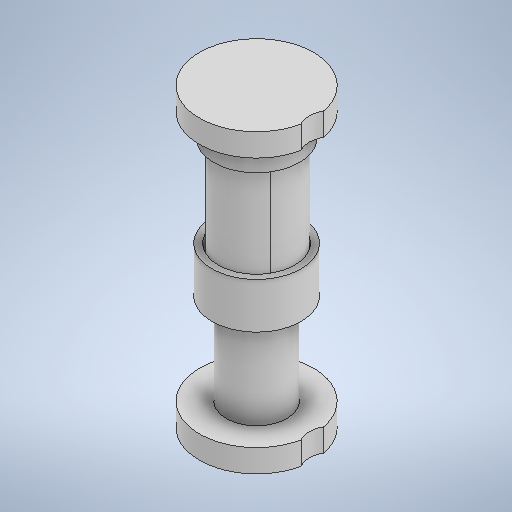
# Autodesk Inventor part: MOULD
Saved by Autodesk Inventor 2026 (Build 300175050, 175E)
## iProperties
Created: 2025-09-13
Part Number: MOULD
Material: Generic
Document SubType Name: Modeling
Designer: Cupri
Density: 1 g/cm^3
Appearance: Default
Author: Cupri
Autodesk Inventor part; units mm, degrees
ref_plane "YZ Plane" through (0, 0, 0) normal (1, 0, 0) x (0, 1, 0)
ref_plane "XZ Plane" through (0, 0, 0) normal (0, 1, 0) x (-1, 0, 0)
ref_plane "XY Plane" through (0, 0, 0) normal (0, 0, 1) x (1, 0, 0)
sketch "Sketch1" plane through (0, 0, 0) normal (0, 1, 0) x (-1, 0, 0)
  circle A0 centre (0, 0) radius 6.75
  circle A1 centre (0, 0) radius 8.25
  dimension "d0" = 13.5
  dimension "d1" = 1.5
  constraints: 2 centre point, 2 coincident
  measures "d0" diameter of A0
  measures "d1" radial gap between concentric circles of A0 A1
extrude "Extrusion1" add sketch "Sketch1" along normal blind 30
sketch "Sketch2" plane through (0, 30, 0) normal (0, 1, 0) x (1, 0, 0)
  circle A0 centre (0, 0) radius 12.5
  dimension "d4" = 25
  constraints: 1 centre point, 1 coincident
  measures "d4" diameter of A0
extrude "Extrusion2" add sketch "Sketch2" along normal blind 5 separate body
sketch "Sketch3" plane through (0, 30, 0) normal (0, -1, 0) x (1, 0, 0)
  line L0 (0, 5) -> (4.3301, 2.5) construction
  line L1 (4.3301, 2.5) -> (4.3301, -2.5) construction
  line L2 (4.3301, -2.5) -> (0, -5) construction
  line L3 (0, -5) -> (-4.3301, -2.5) construction
  line L4 (-4.3301, -2.5) -> (-4.3301, 2.5) construction
  line L5 (-4.3301, 2.5) -> (0, 5) construction
  circle A0 centre (0, 0) radius 6.75 projected
  circle A1 centre (0, 0) radius 1.5 construction
  line L6 (-4.3301, 2.5) -> (-1.1052, -1.0142)
  line L7 (-4.3301, 2.5) -> (0.3257, 1.4642)
  line L8 (0, 5) -> (-1.4309, 0.45)
  line L9 (0, 5) -> (1.4309, 0.45)
  line L10 (4.3301, 2.5) -> (-0.3257, 1.4642)
  line L11 (4.3301, 2.5) -> (1.1052, -1.0142)
  line L12 (4.3301, -2.5) -> (1.1052, 1.0142)
  line L13 (4.3301, -2.5) -> (-0.3257, -1.4642)
  line L14 (0, -5) -> (1.4309, -0.45)
  line L15 (0, -5) -> (-1.4309, -0.45)
  line L16 (-4.3301, -2.5) -> (0.3257, -1.4642)
  line L17 (-4.3301, -2.5) -> (-1.1052, 1.0142)
  point P0 (-1.0179, 1.7631)
  point P1 (-2.0359, 0)
  point P2 (-1.0179, -1.7631)
  point P3 (1.0179, -1.7631)
  point P4 (2.0359, 0)
  point P5 (1.0179, 1.7631)
  dimension "d8" = 3
  dimension "d7" = 5
  constraints: 36 end point, 2 coincident, 39 other
  measures "d7" distance of point (0, 0) L0.start
extrude "Extrusion3" add sketch "Sketch3" along normal blind 25 contours L7 L8 L17 L6 | L17 L8 L7 L10 L9 L12 L11 L14 L13 L16 L15 L6 | L6 L15 L16 L17 | L8 L9 L10 L7 | L16 L13 L14 L15 | L10 L11 L12 L9 | L14 L11 L12 L13 bodies 2
ref_plane "Work Plane2" through (4.3301, 5, 2.5) normal (0.5, 0, -0.8660254) x (-0.8660254, 0, -0.5)
split body "Split2" result two bodies by plane through (4.3301, 5, 2.5) normal (0.5, 0, -0.8660254) bodies 1 first body at (-6.3781, 20, -4.4025)
sketch "Sketch4" plane through (0, 30, 0) normal (0, -1, 0) x (1, 0, 0)
  circle A0 centre (0, 0) radius 8.375
  circle A1 centre (0, 0) radius 9.375
  dimension "d11" = 16.75
  dimension "d12" = 18.75
  constraints: 2 centre point, 2 coincident
  measures "d11" diameter of A0
  measures "d12" diameter of A1
extrude "Extrusion4" add sketch "Sketch4" along normal blind 5 bodies 2
ref_plane "Work Plane3" through (-1.0179, 5, 1.7631) normal (0.8660254, 0, 0.5) x (0.5, 0, -0.8660254)
split body "Split3" result two bodies by plane through (-1.0179, 5, 1.7631) normal (0.8660254, 0, 0.5) bodies 4 first body at (6.4034, 20, 4.3657)
split body "Split4" result two bodies by plane through (-1.0179, 5, 1.7631) normal (0.8660254, 0, 0.5) bodies 3 first body at (5.6812, 20, -5.2713)
sketch "Sketch5" plane through (0, 0, 0) normal (0, -1, 0) x (1, 0, 0)
  circle A0 centre (0, 0) radius 6.625
  line L0 (-4.3301, 2.5) -> (-2.0359, 0) projected
  line L1 (-2.0359, 0) -> (-4.3301, -2.5) projected
  line L2 (-4.3301, -2.5) -> (-1.0179, -1.7631) projected
  line L3 (-1.0179, -1.7631) -> (0, -5) projected
  line L4 (0, -5) -> (1.0179, -1.7631) projected
  line L5 (1.0179, -1.7631) -> (4.3301, -2.5) projected
  line L6 (4.3301, -2.5) -> (2.0359, 0) projected
  line L7 (2.0359, 0) -> (4.3301, 2.5) projected
  line L8 (4.3301, 2.5) -> (1.0179, 1.7631) projected
  line L9 (1.0179, 1.7631) -> (0, 5) projected
  line L10 (0, 5) -> (-1.0179, 1.7631) projected
  line L11 (-1.0179, 1.7631) -> (-4.3301, 2.5) projected
  line L12 (1.1537, -1.9982) -> (0, -5.6667)
  line L13 (0, -5.6667) -> (-1.1537, -1.9982)
  line L14 (-1.1537, -1.9982) -> (-4.9075, -2.8333)
  line L15 (-4.9075, -2.8333) -> (-2.3073, 0)
  line L16 (-2.3073, 0) -> (-4.9075, 2.8333)
  line L17 (-4.9075, 2.8333) -> (-1.1537, 1.9982)
  line L18 (-1.1537, 1.9982) -> (0, 5.6667)
  line L19 (0, 5.6667) -> (1.1537, 1.9982)
  line L20 (1.1537, 1.9982) -> (4.9075, 2.8333)
  line L21 (4.9075, 2.8333) -> (2.3073, 0)
  line L22 (2.3073, 0) -> (4.9075, -2.8333)
  line L23 (4.9075, -2.8333) -> (1.1537, -1.9982)
  dimension "d15" = 13.25
  dimension "d16" = 0.2
  constraints: 24 end point, 1 centre point, 1 coincident, 11 other
  measures "d15" diameter of A0
  measures "d16" distance between parallel lines of L4 L12
extrude "Extrusion5" add sketch "Sketch5" along normal blind 25 separate body contours A0
sketch "Sketch6" plane through (0, -25, 0) normal (0, -1, 0) x (1, 0, 0)
  circle A0 centre (0, 0) radius 12.5
  constraints: 1 centre point, 1 coincident
extrude "Extrusion6" add sketch "Sketch6" along normal blind 5 bodies 9
fillet "Fillet1" radius 0.05 6 edges at (0, 17.5, 5) (4.3301, 17.5, 2.5) (4.3301, 17.5, -2.5) (0, 17.5, -5) (-4.3301, 17.5, -2.5) (-4.3301, 17.5, 2.5)
sketch "Sketch7" plane through (0, 0, 0) normal (0, -1, 0) x (1, 0, 0)
  arc A0 (3.375, -5.8457) -> (5.8457, 3.375) centre (0, 0) ccw projected
  arc A1 (3.375, -5.8457) -> (5.8457, 3.375) centre (0, 0) ccw projected
  circle A2 centre (0, 0) radius 6.75
  circle A3 centre (0, 0) radius 9.75
  arc A4 (4.125, -7.1447) -> (7.1447, 4.125) centre (0, 0) ccw projected
  arc A5 (4.125, -7.1447) -> (7.1447, 4.125) centre (0, 0) ccw projected
  dimension "d22" = 1.5
  constraints: 2 centre point, 2 coincident, 1 concentric
  measures "d22" radial gap between concentric circles of A4 A3
extrude "Extrusion7" add sketch "Sketch7" along normal blind 5 separate body
sketch "Sketch8" plane through (0, 0, 0) normal (0, 1, 0) x (1, 0, 0)
  circle A0 centre (0, 0) radius 9.75 projected
  arc A1 (4.125, 7.1447) -> (-7.1447, 4.125) centre (0, 0) ccw projected
  circle A2 centre (0, 0) radius 8.35
  dimension "d27" = 16.7
  constraints: 1 centre point, 1 coincident
  measures "d27" diameter of A2
extrude "Extrusion8" add sketch "Sketch8" along normal blind 5 bodies 10
sketch "Sketch9" plane through (0, 30, 0) normal (0, -1, 0) x (1, 0, 0)
  arc A0 (5.8457, 3.375) -> (-3.375, 5.8457) centre (0, 0) ccw projected
  circle A1 centre (0, 0) radius 8.375 projected
  line L0 (-4.1749, 2.4655) -> (-1.0179, 1.7631) projected
  line L1 (-1.0179, 1.7631) -> (-0.0477, 4.8483) projected
  arc A2 (0.0477, 4.8483) -> (-0.0477, 4.8483) centre (0, 4.8333) ccw projected
  line L2 (0.0477, 4.8483) -> (1.0179, 1.7631) projected
  line L3 (1.0179, 1.7631) -> (4.1749, 2.4655) projected
  arc A3 (4.2226, 2.3829) -> (4.1749, 2.4655) centre (4.1858, 2.4167) ccw projected
  line L4 (4.2226, 2.3829) -> (2.0359, 0) projected
  line L5 (2.0359, 0) -> (4.2226, -2.3829) projected
  arc A4 (4.1749, -2.4655) -> (4.2226, -2.3829) centre (4.1858, -2.4167) ccw projected
  line L6 (4.1749, -2.4655) -> (1.0179, -1.7631) projected
  line L7 (1.0179, -1.7631) -> (0.0477, -4.8483) projected
  arc A5 (-0.0477, -4.8483) -> (0.0477, -4.8483) centre (0, -4.8333) ccw projected
  line L8 (-0.0477, -4.8483) -> (-1.0179, -1.7631) projected
  line L9 (-1.0179, -1.7631) -> (-4.1749, -2.4655) projected
  arc A6 (-4.2226, -2.3829) -> (-4.1749, -2.4655) centre (-4.1858, -2.4167) ccw projected
  line L10 (-4.2226, -2.3829) -> (-2.0359, 0) projected
  line L11 (-2.0359, 0) -> (-4.2226, 2.3829) projected
  arc A7 (-4.1749, 2.4655) -> (-4.2226, 2.3829) centre (-4.1858, 2.4167) ccw projected
  line L12 (1.1537, 1.9982) -> (0.2385, 4.9083)
  arc A8 (0.2385, 4.9083) -> (-0.2385, 4.9083) centre (0, 4.8333) ccw
  line L13 (-0.2385, 4.9083) -> (-1.1537, 1.9982)
  line L14 (-1.1537, 1.9982) -> (-4.1315, 2.6607)
  arc A9 (-4.1315, 2.6607) -> (-4.37, 2.2476) centre (-4.1858, 2.4167) ccw
  line L15 (-4.37, 2.2476) -> (-2.3073, 0)
  line L16 (-2.3073, 0) -> (-4.37, -2.2476)
  arc A10 (-4.37, -2.2476) -> (-4.1315, -2.6607) centre (-4.1858, -2.4167) ccw
  line L17 (-4.1315, -2.6607) -> (-1.1537, -1.9982)
  line L18 (-1.1537, -1.9982) -> (-0.2385, -4.9083)
  arc A11 (-0.2385, -4.9083) -> (0.2385, -4.9083) centre (0, -4.8333) ccw
  line L19 (0.2385, -4.9083) -> (1.1537, -1.9982)
  line L20 (1.1537, -1.9982) -> (4.1315, -2.6607)
  arc A12 (4.1315, -2.6607) -> (4.37, -2.2476) centre (4.1858, -2.4167) ccw
  line L21 (4.37, -2.2476) -> (2.3073, 0)
  line L22 (2.3073, 0) -> (4.37, 2.2476)
  arc A13 (4.37, 2.2476) -> (4.1315, 2.6607) centre (4.1858, 2.4167) ccw
  line L23 (4.1315, 2.6607) -> (1.1537, 1.9982)
  circle A14 centre (0, 0) radius 6.65
  dimension "d30" = 0.2
  dimension "d31" = 13.3
  constraints: 24 end point, 12 point on circle, 7 centre point, 1 coincident, 17 other
  measures "d30" distance between parallel lines of L2 L12
  measures "d31" diameter of A14
extrude "Extrusion9" add sketch "Sketch9" along normal blind 5 separate body contours A14
sketch "Sketch10" plane through (0, -30, 0) normal (0, -1, 0) x (1, 0, 0)
  circle A0 centre (0, 0) radius 12.5 projected
  circle A1 centre (0, 0) radius 9.75 projected
  arc A2 (12.2474, 2.5) -> (12.2474, -2.5) centre (16.5776, 0) ccw
  dimension "d34" = 5
  dimension "d35" = 5
  dimension "d36" = 0
  constraints: 4 point on circle, 1 centre point
  measures "d34" distance of A0.end A0.start
  measures "d35" radius of A2
  measures "d36" vertical distance of point (0, 0) A2.centre
extrude "Extrusion10" cut sketch "Sketch10" against normal through all contours A0 A2 picked at (11.9033, 0) bodies 9 2
body "Solid2"
body "Solid12"
body "Solid13"
body "Solid15"
body "Solid8"
body "Solid9"
body "Solid10"
body "Solid11"
